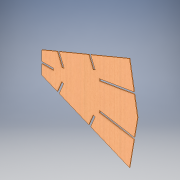
# Autodesk Inventor part: refbot
Saved by Autodesk Inventor 2019 (Build 230136000, 136)
## iProperties
Created: 2019-01-23
Part Number: refbot
Material: Wood (Cherry)
Document SubType Name: Modeling
Designer: gaincarlo
Density: 0.63 g/cm^3
Appearance: Cherry - Natural Low Gloss
Author: gaincarlo
Autodesk Inventor part; units mm, degrees
ref_plane "YZ Plane" through (0, 0, 0) normal (1, 0, 0) x (0, 1, 0)
ref_plane "XZ Plane" through (0, 0, 0) normal (0, 1, 0) x (-1, 0, 0)
ref_plane "Work Plane1" through (0, 0, 0) normal (0, 0, 1) x (1, 0, 0)
sketch "Sketch1" plane through (0, 0, 0) normal (0, 0, 1) x (1, 0, 0)
  line L0 (-79.5271, 221.8978) -> (-38.5876, 0.7641) construction
  line L1 (-214.8536, 60) -> (-51.8859, 87.6696) projected
  line L2 (-53.5598, 97.5285) -> (-216.5275, 69.8589) projected
  line L3 (-216.5275, 69.8589) -> (-214.8536, 60) projected
  line L4 (-265.8796, 142.5897) -> (-244.8522, 91.8249) projected
  line L5 (-235.6134, 95.6518) -> (-256.6408, 146.4165) projected
  line L6 (-235.6134, 95.6518) -> (-244.8522, 91.8249) projected
  line L7 (-413.7003, -81.3604) -> (-404.4616, -85.1872) construction
  line L8 (-392.6729, -30.5956) -> (-413.7003, -81.3604) projected
  line L9 (-404.4616, -85.1872) -> (-383.4341, -34.4224) projected
  line L10 (-244.8727, -91.8744) -> (-265.9001, -142.6392) projected
  line L11 (-265.9001, -142.6392) -> (-256.6613, -146.466) construction
  line L12 (-256.6613, -146.466) -> (-235.6339, -95.7013) projected
  line L13 (-486.3009, 5) -> (-486.3009, -5) construction
  line L14 (-486.3009, -5) -> (-431.3536, -5) projected
  line L15 (-431.3536, 5) -> (-486.3009, 5) projected
  line L16 (-431.3536, 5) -> (-431.3536, -5) projected
  line L17 (-411.8071, 76.7896) -> (-402.5683, 80.6164) construction
  line L18 (-411.8071, 76.7896) -> (-390.7796, 26.0248) projected
  line L19 (-381.5408, 29.8516) -> (-402.5683, 80.6164) projected
  line L20 (-390.7796, 26.0248) -> (-381.5408, 29.8516) projected
  line L21 (-256.6408, 146.4165) -> (-265.8796, 142.5897) construction
  line L22 (-167.233, 78.2284) -> (-53.5598, 97.5285) projected
  line L23 (-51.8859, 87.6696) -> (-165.5591, 68.3695) projected
  line L24 (-53.5598, 97.5285) -> (-51.8859, 87.6696) construction
  line L25 (-51.7174, -86.6773) -> (-214.6851, -59.0077) projected
  line L26 (-51.7174, -86.6773) -> (-53.3913, -96.5362) construction
  line L27 (-216.359, -68.8666) -> (-53.3913, -96.5362) projected
  line L28 (-214.6851, -59.0077) -> (-216.359, -68.8666) projected
  line L29 (-392.6729, -30.5956) -> (-383.4341, -34.4224) projected
  line L30 (-244.8727, -91.8744) -> (-235.6339, -95.7013) projected
  line L31 (-481.3536, 5) -> (-431.3536, 5) projected
  line L32 (-486.3009, -51.2882) -> (-413.7003, -81.3604)
  line L33 (-486.3009, -51.2882) -> (-486.3009, -5)
  line L34 (-486.3009, 5) -> (-486.3009, 51.2882)
  line L35 (-256.6408, 146.4165) -> (-74.6586, 221.796)
  line L36 (-37.0008, 0) -> (-51.8859, 87.6696)
  line L37 (-53.5598, 97.5285) -> (-74.6586, 221.796)
  line L38 (-74.6586, -221.796) -> (-53.3913, -96.5362)
  line L39 (-51.7174, -86.6773) -> (-37.0008, 0)
  line L40 (-404.4616, -85.1872) -> (-265.8796, -142.5897)
  line L41 (-256.6408, -146.4165) -> (-74.6586, -221.796)
  line L42 (-411.8071, 76.7896) -> (-413.7003, 81.3604)
  line L43 (-402.5683, 80.6164) -> (-404.4616, 85.1872)
  line L44 (-486.3009, 51.2882) -> (-413.7003, 81.3604)
  line L45 (-404.4616, 85.1872) -> (-265.8796, 142.5897)
  point P0 (0, 0)
  constraints: 40 end point, 9 collinear, 3 parallel, 2 perpendicular, 2 point on line
extrude "Extrusion1" add sketch "Sketch1" along normal blind 3
body "Solid1"
